Autodesk Fusion 360 part; units mm, degrees
note: some values were not read from the file. Set by a fixed rule: the direction of a hole.
(part 2 of 4)
sketch "草图3" plane through (0, 0, 16.2) normal (0, 0, 1) x (-1, 0, 0)
  line L0 (-5, -22) -> (0, -17)
  line L1 (0, -17) -> (0, -5)
  line L2 (0, -5) -> (-5, 0)
  line L3 (-5, 0) -> (-17, 0)
  line L4 (-17, 0) -> (-22, -5)
  line L5 (-22, -5) -> (-22, -17)
  line L6 (-22, -17) -> (-17, -22)
  line L7 (-17, -22) -> (-5, -22)
  circle A0 centre (-11, -11) radius 9
  dimension "d13" = 18
  dimension "d14" = 11
  dimension "d15" = 11
  measures "d13" diameter of A0
  measures "d14" distance of L7 A0.centre
  measures "d15" distance of L5 A0.centre
extrude "拉伸3" add sketch "草图3" along normal blind 5.5 contours A0
fillet "圆角4" radius 1 1 edges at (19.3909, 7.7455, 16.2)
chamfer "倒角1" distance 2 angle 45 8 edges at (11, 0, 16.2) (19.5, 2.5, 16.2) (22, 11, 16.2) (19.5, 19.5, 16.2) (2.5, 2.5, 16.2) (0, 11, 16.2) (2.5, 19.5, 16.2) (11, 22, 16.2)
sketch "草图4" plane through (0, 0, 0) normal (0, 0, -1) x (1, 0, 0)
  arc A0 (17, -22) -> (22, -17) centre (17, -17) ccw
  line L0 (22, -17) -> (22, -5)
  arc A1 (22, -5) -> (17, 0) centre (17, -5) ccw
  line L1 (17, 0) -> (5, 0)
  arc A2 (5, 0) -> (0, -5) centre (5, -5) ccw
  line L2 (0, -5) -> (0, -17)
  arc A3 (0, -17) -> (5, -22) centre (5, -17) ccw
  line L3 (5, -22) -> (17, -22)
  circle A4 centre (4.75, -17) radius 1.2
  circle A5 centre (17.25, -17) radius 1.2
  dimension "d23" = 2.4
  dimension "d24" = 2.4
  dimension "d25" = 12.5
  dimension "d26" = 4.75
  dimension "d27" = 5
  measures "d23" diameter of A4
  measures "d24" diameter of A5
  measures "d25" distance of A4.centre A5.centre
  measures "d26" distance of L2 A4.centre
  measures "d27" distance of L3 A4.centre
extrude "拉伸4" cut sketch "草图4" against normal blind 5 contours A4 | A5
sketch "草图5" plane through (0, 0, 0) normal (0, 0, -1) x (1, 0, 0)
  circle A0 centre (4.75, -17) radius 1.2
  circle A1 centre (17.25, -17) radius 1.2
  arc A2 (17, -22) -> (22, -17) centre (17, -17) ccw
  line L0 (22, -17) -> (22, -5)
  arc A3 (22, -5) -> (17, 0) centre (17, -5) ccw
  line L1 (17, 0) -> (5, 0)
  arc A4 (5, 0) -> (0, -5) centre (5, -5) ccw
  line L2 (0, -5) -> (0, -17)
  arc A5 (0, -17) -> (5, -22) centre (5, -17) ccw
  line L3 (5, -22) -> (17, -22)
  circle A6 centre (11, -14) radius 3.25
  dimension "d30" = 6.5
  dimension "d33" = 8
  measures "d30" diameter of A6
  measures "d33" distance of L3 A6.centre
extrude "拉伸5" add sketch "草图5" along normal blind 3 contours A6

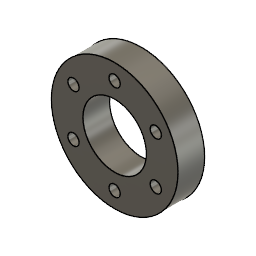
design "输出轴垫块---2"
part number: 2026-07-22-15-46-42-042
Autodesk Fusion 360 part; units mm, degrees
sketch "草图1" plane through (0, 0, 0) normal (0, 0, 1) x (1, 0, 0)
  circle A0 centre (6.115, -10.5915) radius 1.7
  circle A1 centre (-12.23, 0) radius 1.7
  arc A2 (-10.145, 12.6301) -> (-10.3229, 9.3593) centre (-8.7673, 10.9149) ccw
  circle A3 centre (6.115, 10.5915) radius 1.7
  arc A4 (-1.5064, -8.2546) -> (-2.6915, -5.6961) centre (-3.6314, -7.6852) ccw
  arc A5 (-2.9439, 13.6195) -> (-5.8655, 15.1009) centre (-5.0689, 13.0501) ccw
  line L0 (13.2668, -4.2603) -> (7.9019, -2.8228)
  line L1 (-6.3955, 5.4319) -> (-10.3229, 9.3593)
  circle A6 centre (11.6913, 6.75) radius 1.6
  line L2 (-2.9439, 13.6195) -> (-1.5064, 8.2547)
  arc A7 (6.2787, -0.5171) -> (6.2787, 0.5171) centre (0, 0) ccw
  arc A8 (16.0105, 2.4708) -> (13.2668, 4.2603) centre (13.8362, 2.1352) ccw
  arc A9 (-5.8655, 15.1009) -> (-10.145, 12.6301) centre (0, 0) ccw
  line L3 (7.9019, 2.8227) -> (13.2668, 4.2603)
  circle A10 centre (11.6913, -6.75) radius 1.6
  arc A11 (13.2668, -4.2603) -> (16.0105, -2.4708) centre (13.8362, -2.1352) ccw
  arc A12 (-10.145, -12.6301) -> (-5.8655, -15.1009) centre (0, 0) ccw
  arc A13 (-10.3229, -9.3593) -> (-10.145, -12.6301) centre (-8.7673, -10.9149) ccw
  arc A14 (-3.5872, -5.179) -> (-6.3955, -5.4319) centre (-4.8399, -6.9875) ccw
  circle A15 centre (0, 13.5) radius 1.6
  circle A16 centre (-11.6913, -6.75) radius 1.6
  circle A17 centre (0, 0) radius 4.75
  arc A18 (-2.6915, 5.6961) -> (-3.5872, 5.179) centre (0, 0) ccw
  circle A19 centre (-11.6913, 6.75) radius 1.6
  arc A20 (6.2787, -0.5171) -> (7.9019, -2.8228) centre (8.4713, -0.6977) ccw
  arc A21 (-6.3955, 5.4319) -> (-3.5872, 5.179) centre (-4.8399, 6.9875) ccw
  arc A22 (-3.5872, -5.179) -> (-2.6915, -5.6961) centre (0, 0) ccw
  circle A23 centre (0, -13.5) radius 1.6
  arc A24 (-2.6915, 5.6961) -> (-1.5064, 8.2547) centre (-3.6314, 7.6852) ccw
  circle A25 centre (0, 0) radius 18
  arc A26 (7.9019, 2.8227) -> (6.2787, 0.5171) centre (8.4713, 0.6977) ccw
  line L4 (-1.5064, -8.2546) -> (-2.9439, -13.6195)
  line L5 (-10.3229, -9.3593) -> (-6.3955, -5.4319)
  arc A27 (16.0105, -2.4708) -> (16.0105, 2.4708) centre (0, 0) ccw
  arc A28 (-5.8655, -15.1009) -> (-2.9439, -13.6195) centre (-5.0689, -13.0501) ccw
  dimension "d3" = 36
  dimension "d4" = 3.2
  constraint equal A6 A15
  constraint equal A6 A10
  constraint equal A10 A23
  constraint equal A16 A23
  constraint equal A16 A19
  measures "d3" diameter of A25
  measures "d4" diameter of A15
extrude "拉伸1" add sketch "草图1" along normal blind 7.6 contours A0 | A1 | A2 A5 L1 L2 A9 A18 A21 A24 | A3 | A4 A12 A13 A14 A22 L4 L5 A28 | L0 A7 A8 L3 A11 A20 A26 A27 | A25
sketch "草图2" plane through (0, 0, 7.6) normal (0, 0, 1) x (1, 0, 0)
  circle A0 centre (11.6913, -6.75) radius 1.6
  circle A1 centre (11.6913, 6.75) radius 1.6
  circle A2 centre (-11.6913, 6.75) radius 1.6
  circle A3 centre (0, 13.5) radius 1.6
  circle A4 centre (-11.6913, -6.75) radius 1.6
  circle A5 centre (0, 0) radius 4.75
  circle A6 centre (0, -13.5) radius 1.6
  circle A7 centre (0, 0) radius 18
  circle A8 centre (0, 0) radius 9
  dimension "d5" = 18
  constraint coincident A5.centre A7.centre
  measures "d5" diameter of A8
extrude "拉伸2" cut sketch "草图2" against normal blind 20 contours A8

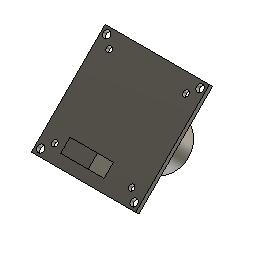
design "New Camera"
part number: 2026-07-08-15-06-55-000
Autodesk Fusion 360 part; units mm, degrees
sketch "sketch 1014" plane through (0, -331.5766, 331.5766) normal (0, -0.707107, 0.707107) x (1, 0, 0)
  line L0 (19, 44) -> (19, 82)
  line L1 (19, 82) -> (-19, 82)
  line L2 (-19, 82) -> (-19, 44)
  line L3 (-19, 44) -> (19, 44)
  circle A0 centre (14, 77) radius 1
  circle A1 centre (17, 80) radius 1.25
  circle A2 centre (-14, 49) radius 1
  circle A3 centre (-17, 80) radius 1.25
  circle A4 centre (-14, 77) radius 1
  circle A5 centre (17, 46) radius 1.25
  circle A6 centre (14, 49) radius 1
  circle A7 centre (-17, 46) radius 1.25
extrude "拉伸1" add sketch "sketch 1014" along normal blind 1.6
sketch "草图1" plane through (0, -331.5766, 331.5766) normal (0, 0.707107, -0.707107) x (-1, 0, 0)
  line L0 (-19, 82) -> (-19, 44)
  line L1 (-19, 44) -> (19, 44)
  line L2 (19, 44) -> (19, 82)
  line L3 (19, 82) -> (-19, 82)
  circle A0 centre (-17, 46) radius 1.25
  circle A1 centre (-14, 77) radius 1
  circle A2 centre (14, 77) radius 1
  circle A3 centre (17, 80) radius 1.25
  circle A4 centre (17, 46) radius 1.25
  circle A5 centre (-14, 49) radius 1
  circle A6 centre (-17, 80) radius 1.25
  circle A7 centre (14, 49) radius 1
  line L4 (-19, 82) -> (19, 44) construction
  line L5 (19, 82) -> (-19, 44) construction
  line L6 (-7, 70) -> (7, 70)
  line L7 (7, 70) -> (7, 56)
  line L8 (7, 56) -> (-7, 56)
  line L9 (-7, 56) -> (-7, 70)
  line L10 (-7, 70) -> (7, 56) construction
  line L11 (7, 70) -> (-7, 56) construction
  line L12 (-7, 63) -> (7, 63) construction
  line L13 (-7, 65.15) -> (-8.85, 65.15)
  arc A8 (-8.85, 65.15) -> (-8.85, 60.85) centre (-8.85, 63) ccw
  line L14 (-8.85, 60.85) -> (-7, 60.85)
  line L15 (0, 70) -> (0, 56) construction
  arc A9 (8.85, 60.85) -> (8.85, 65.15) centre (8.85, 63) ccw
  line L16 (7, 65.15) -> (8.85, 65.15)
  line L17 (8.85, 60.85) -> (7, 60.85)
  point P0 (0, 63)
  point P1 (0, 63)
  point P2 (-11, 63)
  dimension "d359" = 14
  dimension "d360" = 4.3
  dimension "d362" = 11
  constraint coincident L0.start L3.end
  constraint coincident L1.end L2.start
  constraint coincident L2.end L3.start
  constraint coincident L0.end L1.start
  constraint midpoint L4 P1
  constraint horizontal L6
  constraint perpendicular L6 L7
  constraint parallel L6 L8
  constraint parallel L7 L9
  constraint coincident L10 P1
  constraint coincident L11 P1
  constraint coincident P1 P0
  constraint equal L6 L9
  constraint midpoint L9 L12.start
  constraint midpoint L7 L12.end
  constraint coincident L9 L13.start
  constraint perpendicular L9 L13
  constraint tangent L13 A8
  constraint coincident L9 L14.end
  constraint tangent A8 L14
  constraint perpendicular L9 L14
  constraint symmetric L12 L13.start L14.end
  constraint midpoint A8 P2
  constraint midpoint L6 L15.start
  constraint midpoint L8 L15.end
  constraint symmetric L13.start L15 L16.start
  constraint symmetric L13.end L15 A9.end
  constraint symmetric A8.end L15 A9.start
  constraint symmetric A8 L15 A9
  constraint symmetric L14.end L15 L17.end
  measures "d359" distance of L6.end L7.end
  measures "d360" distance of L13 L14
  measures "d362" distance of P1 P2
extrude "拉伸2" add sketch "草图1" along normal blind 3.5 contours L6 L7 L8 L9 | L9 L13 A8 L14 | L7 A9 L16 L17
sketch "草图2" plane through (0, -329.1018, 329.1018) normal (0, 0.707107, -0.707107) x (-1, 0, 0)
  line L0 (-7, 65.15) -> (-8.85, 65.15)
  arc A0 (-8.85, 65.15) -> (-8.85, 60.85) centre (-8.85, 63) ccw
  line L1 (-8.85, 60.85) -> (-7, 60.85)
  line L2 (-7, 60.85) -> (-7, 56)
  line L3 (-7, 56) -> (7, 56)
  line L4 (7, 56) -> (7, 60.85)
  line L5 (7, 60.85) -> (8.85, 60.85)
  arc A1 (8.85, 60.85) -> (8.85, 65.15) centre (8.85, 63) ccw
  line L6 (8.85, 65.15) -> (7, 65.15)
  line L7 (7, 65.15) -> (7, 70)
  line L8 (7, 70) -> (-7, 70)
  line L9 (-7, 70) -> (-7, 65.15)
  line L10 (0, 70) -> (0, 56) construction
  circle A2 centre (0, 63) radius 7
  dimension "d365" = 14
  constraint midpoint L8 L10.start
  constraint midpoint L3 L10.end
  constraint midpoint L10 A2.centre
  measures "d365" diameter of A2
extrude "拉伸3" add sketch "草图2" along normal blind 10.6 contours A2
sketch "草图3" plane through (1.3279, -320.4832, 322.7296) normal (0, 0.707107, -0.707107) x (-1, 0, 0)
  circle A0 centre (1.3279, 61.4116) radius 8.5
  circle A1 centre (1.3279, 61.4116) radius 7 construction
  dimension "d369" = 17
  constraint coincident A0.centre A1.centre
  measures "d369" diameter of A0
extrude "拉伸4" add sketch "草图3" along normal blind 7.3
sketch "草图4" plane through (0, -332.708, 332.708) normal (0, -0.707107, 0.707107) x (1, 0, 0)
  line L0 (-19, 44) -> (19, 44)
  line L1 (19, 44) -> (19, 82)
  line L2 (19, 82) -> (-19, 82)
  line L3 (-19, 82) -> (-19, 44)
  circle A0 centre (14, 49) radius 1
  circle A1 centre (-14, 77) radius 1
  circle A2 centre (17, 46) radius 1.25
  circle A3 centre (-17, 80) radius 1.25
  circle A4 centre (-14, 49) radius 1
  circle A5 centre (-17, 46) radius 1.25
  circle A6 centre (17, 80) radius 1.25
  circle A7 centre (14, 77) radius 1
  line L4 (-5, 52.3) -> (5, 52.3)
  line L5 (5, 52.3) -> (5, 47.5)
  line L6 (5, 47.5) -> (-5, 47.5)
  line L7 (-5, 47.5) -> (-5, 52.3)
  line L8 (0, 44) -> (0, 52.3) construction
  line L9 (-19, 44) -> (19, 44)
  dimension "d1" = 3.5
  dimension "d2" = 4.8
  dimension "d3" = 10
  constraint horizontal L4
  constraint vertical L5
  constraint horizontal L6
  constraint vertical L7
  constraint midpoint L0 L8.start
  constraint midpoint L4 L8.end
  constraint vertical L8
  measures "d1" distance of L6 L9
  measures "d2" distance of L4.start L6.end
  measures "d3" distance of L4.start L4.end
extrude "拉伸5" add sketch "草图4" along normal blind 8.2 contours L4 L5 L6 L7

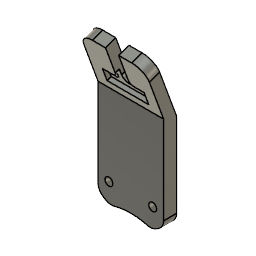
design "Maker Arm 摄像头支架-UW"
part number: 2026-08-07-11-14-49-423
Autodesk Fusion 360 part; units mm, degrees
sketch "草图2" plane through (0, 0, 0) normal (1, 0, 0) x (0, 1, 0)
  line L0 (-6, 73.2538) -> (-6, 0)
  line L1 (0, 71.388) -> (0, 0)
  line L2 (-6, 0) -> (0, 0)
  line L3 (0, 71.388) -> (-9.852, 98.4563)
  line L4 (-9.852, 98.4563) -> (-14.5505, 96.7462)
  line L5 (-14.5505, 96.7462) -> (-6, 73.2538)
  point P0 (-10.2753, 85)
  dimension "d70" = 6
  dimension "d71" = 5
  dimension "d72" = 25
  dimension "d73" = 160
  dimension "d74" = 85
  constraint vertical L0
  constraint vertical L1
  constraint perpendicular L1 L2
  constraint coincident L1.end L2.end
  constraint perpendicular L3 L4
  constraint perpendicular L4 L5
  constraint midpoint L5 P0
  measures "d70" distance of L0.end L1.end
  measures "d71" distance of L3.end L4.end
  measures "d72" distance of L0.start L4.end
  measures "d73" angle of L0 L5
  measures "d74" distance of L2 P0
extrude "拉伸2" add sketch "草图2" along normal mid plane 30
sketch "草图12" plane through (0, -6, 0) normal (0, -1, 0) x (1, 0, 0)
  line L0 (-15, 0) -> (15, 0)
  line L1 (15, 0) -> (15, 73.2538)
  line L2 (15, 73.2538) -> (-15, 73.2538)
  line L3 (-15, 73.2538) -> (-15, 0)
  circle A0 centre (0, 0) radius 28.5
  circle A1 centre (-10, 36) radius 1.8
  circle A2 centre (10, 36) radius 1.8
  line L4 (0, 0) -> (0, 28.5) construction
  dimension "d92" = 57
  dimension "d93" = 3.6
  dimension "d94" = 36
  dimension "d95" = 20
  constraint coincident A0.centre L4.start
  constraint coincident A0 L4.end
  constraint perpendicular L0 L4
  constraint symmetric A1.centre A2.centre L4
  constraint equal A1 A2
  measures "d92" diameter of A0
  measures "d93" diameter of A1
  measures "d94" vertical distance of A0.centre A1.centre
  measures "d95" distance of A1.centre A2.centre
extrude "拉伸13" cut sketch "草图12" against normal up to surface (6 mm away) contours L0 L1 L3 A0 | A1 | A2 picked at (0, 9.5)
chamfer "倒角5" distance 6 angle 45 2 edges at (-15, -3, 24.2332) (15, -3, 24.2332)
fillet "圆角2" radius 5 4 edges at (-9.5942, -3, 26.8366) (9.5942, -3, 26.8366) (-15, -3, 30.2332) (15, -3, 30.2332)
sketch "草图13" plane through (0, 22.9437, 8.3508) normal (0, 0.939693, 0.34202) x (-1, 0, 0)
  line L0 (15, 95.8882) -> (-15, 95.8882)
  line L1 (-15, 95.8882) -> (-15, 67.0828)
  line L2 (-15, 67.0828) -> (15, 67.0828)
  line L3 (15, 67.0828) -> (15, 95.8882)
  line L4 (-3, 95.8882) -> (-3, 79.8882)
  arc A0 (-3, 79.8882) -> (3, 79.8882) centre (0, 79.8882) ccw
  line L5 (3, 79.8882) -> (3, 95.8882)
  line L6 (-6.25, 77.8882) -> (6.25, 77.8882) construction
  line L7 (0, 95.8882) -> (0, 77.8882) construction
  circle A1 centre (-6.25, 77.8882) radius 1.2
  circle A2 centre (6.25, 77.8882) radius 1.2
  line L8 (-11, 72.3882) -> (11, 72.3882) construction
  line L9 (11, 72.3882) -> (11, 94.3882) construction
  line L10 (11, 94.3882) -> (-11, 94.3882) construction
  line L11 (-11, 94.3882) -> (-11, 72.3882) construction
  line L12 (-11, 72.3882) -> (11, 94.3882) construction
  line L13 (11, 72.3882) -> (-11, 94.3882) construction
  point P0 (0, 83.3882)
  dimension "d103" = 3
  dimension "d105" = 2.4
  dimension "d106" = 12.5
  dimension "d107" = 2
  dimension "d109" = 22
  dimension "d110" = 3.5
  dimension "d111" = 12.5
  constraint coincident L0 L4.start
  constraint perpendicular L0 L4
  constraint tangent L4 A0
  constraint tangent A0 L5
  constraint perpendicular L0 L5
  constraint horizontal L6
  constraint midpoint L0 L7.start
  constraint midpoint L6 L7.end
  constraint coincident L6.start A1.centre
  constraint coincident L6.end A2.centre
  constraint equal A1 A2
  constraint vertical L7
  constraint coincident A0.centre L7
  constraint coincident L0 L5.end
  constraint horizontal L8
  constraint perpendicular L8 L9
  constraint parallel L8 L10
  constraint parallel L9 L11
  constraint coincident L12 P0
  constraint coincident L13 P0
  constraint coincident L7 P0
  constraint equal L10 L11
  measures "d103" radius of A0
  measures "d105" diameter of A1
  measures "d106" distance of L6.start L6.end
  measures "d107" distance of A0.centre L6
  measures "d109" distance of L8.start L8.end
  measures "d110" distance of A0.centre P0
  measures "d111" distance of L7.start P0
extrude "拉伸14" cut sketch "草图13" against normal up to surface (5 mm away) contours L0 L4 A0 L5 | A1 | A2
sketch "草图15" plane through (0, 18.2452, 6.6407) normal (0, -0.939693, -0.34202) x (1, 0, 0)
  line L0 (3, 95.8882) -> (3, 79.8882)
  arc A0 (-3, 79.8882) -> (3, 79.8882) centre (0, 79.8882) ccw
  line L1 (-3, 79.8882) -> (-3, 95.8882)
  line L2 (-3, 95.8882) -> (-15, 95.8882)
  line L3 (-15, 95.8882) -> (-15, 70.8882)
  line L4 (-15, 70.8882) -> (15, 70.8882)
  line L5 (15, 70.8882) -> (15, 95.8882)
  line L6 (15, 95.8882) -> (3, 95.8882)
  circle A1 centre (-6.25, 77.8882) radius 1.2
  circle A2 centre (6.25, 77.8882) radius 1.2
  line L7 (-9.5, 80.9882) -> (9.5, 80.9882)
  line L8 (9.5, 80.9882) -> (9.5, 74.7882)
  line L9 (9.5, 74.7882) -> (-9.5, 74.7882)
  line L10 (-9.5, 74.7882) -> (-9.5, 80.9882)
  line L11 (-9.5, 77.8882) -> (9.5, 77.8882) construction
  line L12 (0, 80.9882) -> (0, 74.7882) construction
  dimension "d120" = 6.2
  dimension "d121" = 19
  constraint horizontal L7
  constraint vertical L8
  constraint horizontal L9
  constraint vertical L10
  constraint midpoint L10 L11.start
  constraint midpoint L8 L11.end
  constraint midpoint L7 L12.start
  constraint midpoint L9 L12.end
  constraint coincident A1.centre L11
  constraint symmetric A1.centre A2.centre L12
  measures "d120" distance of L7.start L9.end
  measures "d121" distance of L8.end L9.end
extrude "拉伸16" cut sketch "草图15" against normal blind 2 contours L0 A0 L1 L7 L8 L9 L10
fillet "圆角4" radius 2 2 edges at (-3, -8.5147, 83.0868) (3, -8.5147, 83.0868)
fillet "圆角4" radius 6 2 edges at (-15, -12.2013, 97.6012) (15, -12.2013, 97.6012)

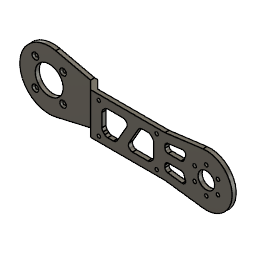
design "L2侧臂-2"
part number: 2026-08-10-10-33-43-885
Autodesk Fusion 360 part; units mm, degrees
sketch "草图1" plane through (0, 0, 0) normal (0, 0, 1) x (1, 0, 0)
  line L0 (0, -20) -> (160, -20)
  arc A0 (160, -20) -> (160, 20) centre (160, 0) ccw
  line L1 (160, 20) -> (0, 20)
  arc A1 (0, 20) -> (0, -20) centre (0, 0) ccw
  line L2 (0, 0) -> (160, 0) construction
  circle A2 centre (0, 0) radius 28.5
  circle A3 centre (160, 0) radius 25
  circle A4 centre (160, 0) radius 8
  circle A5 centre (160, 0) radius 13 construction
  circle A6 centre (160, 13) radius 1.65
  circle A7 centre (148.7417, 6.5) radius 1.65
  circle A8 centre (148.7417, -6.5) radius 1.65
  circle A9 centre (160, -13) radius 1.65
  circle A10 centre (171.2583, -6.5) radius 1.65
  circle A11 centre (171.2583, 6.5) radius 1.65
  line L3 (6.4228, 27.7668) -> (40, 20)
  line L4 (6.4228, -27.7668) -> (40, -20)
  line L5 (156.7702, 24.7905) -> (120, 20)
  line L6 (120, -20) -> (156.7702, -24.7905)
  circle A12 centre (0, 0) radius 19 construction
  circle A13 centre (-13.435, 13.435) radius 1.65
  circle A14 centre (-13.435, -13.435) radius 1.65
  circle A15 centre (13.435, -13.435) radius 1.65
  circle A16 centre (13.435, 13.435) radius 1.65
  line L7 (-13.435, 13.435) -> (0, 0) construction
  line L8 (0, 0) -> (0, 32.5193) construction
  circle A17 centre (0, 0) radius 13.5
  dimension "d1" = 160
  dimension "d2" = 16
  dimension "d3" = 26
  dimension "d4" = 3.3
  dimension "d6" = 360
  dimension "d9" = 57
  dimension "d11" = 40
  dimension "d13" = 20
  dimension "d15" = 38
  dimension "d16" = 20
  dimension "d17" = 3.3
  dimension "d19" = 360
  dimension "d20" = 45
  dimension "d21" = 27
  dimension "d75" = 50
  dimension "d76" = 40
  dimension "d77" = 40
  constraint tangent L0 A0
  constraint tangent A0 L1
  constraint parallel L0 L1
  constraint horizontal L2
  constraint coincident A1.centre L2.start
  constraint concentric A0 A3
  constraint concentric A0 A4
  constraint concentric A0 A5
  constraint coincident A5 A6.centre
  constraint vertical A6.centre A9.centre
  constraint coincident A2 L3.start
  constraint coincident L1 L3.end
  constraint coincident A2 L4.start
  constraint coincident L0 L4.end
  constraint tangent A2 L4
  constraint coincident A3 L5.start
  constraint coincident L1 L5.end
  constraint coincident A3 L6.end
  constraint tangent A3 L5
  constraint tangent A3 L6
  constraint coincident L0 L6.start
  constraint concentric A1 A12
  constraint vertical L0.start L1.end
  constraint tangent A2 L3
  constraint coincident A12 A13.centre
  constraint coincident A13.centre L7.start
  constraint perpendicular L2 L8
  constraint concentric A12 A17
  constraint equal L3 L4
  measures "d1" distance of A0.end L1.end
  measures "d2" diameter of A4
  measures "d3" diameter of A5
  measures "d4" diameter of A6
  measures "d9" diameter of A2
  measures "d11" horizontal distance of A1.centre L3.end
  measures "d13" radius of A0
  measures "d15" diameter of A12
  measures "d16" radius of A1
  measures "d17" diameter of A13
  measures "d20" angle of L7 L8
  measures "d21" diameter of A17
  measures "d75" diameter of A3
  measures "d76" horizontal distance of A0.centre L5.end
  measures "d77" horizontal distance of A0.centre L6.start
extrude "拉伸1" add sketch "草图1" along normal blind 12 contours L0 L1 A2 A3 | L0 A2 L4 | L0 A3 L6 | L0 L1 A1 A2 A13 A14 | L0 L1 A1 A2 A13 A14 | L0 A0 L1 A3 | L0 A0 L1 A3 | L1 A2 L3 | L1 A3 L5
sketch "草图2" plane through (0, 20, 0) normal (0, 1, 0) x (-1, 0, 0)
  line L0 (-120, 0) -> (-40, 0)
  line L1 (-40, 0) -> (-40, 12)
  line L2 (-40, 12) -> (-120, 12)
  line L3 (-120, 12) -> (-120, 0)
  line L4 (29.704, 4) -> (-40, 4)
  line L5 (-40, 4) -> (-40, 12)
  line L6 (-40, 12) -> (29.704, 12)
  line L7 (29.704, 12) -> (29.704, 4)
  line L8 (-120, 0) -> (-190, 0)
  line L9 (-190, 0) -> (-190, 8)
  line L10 (-190, 8) -> (-120, 8)
  line L11 (-120, 8) -> (-120, 0)
  line L12 (-40, 4) -> (-48, 12)
  line L13 (-43.0711, 0) -> (-51.0711, 8)
  line L14 (-51.0711, 8) -> (-120, 8)
  dimension "d24" = 8
  dimension "d25" = 8
  dimension "d26" = 45
  dimension "d27" = 5
  constraint horizontal L4
  constraint vertical L5
  constraint horizontal L6
  constraint vertical L7
  constraint coincident L1.end L2.start
  constraint horizontal L8
  constraint vertical L9
  constraint horizontal L10
  constraint vertical L11
  constraint coincident L0.start L3.end
  constraint coincident L2 L12.end
  constraint coincident L0 L13.start
  constraint parallel L12 L13
  constraint horizontal L14
  measures "d24" distance of L8.end L9.end
  measures "d25" distance of L4.start L6.end
  measures "d26" angle of L0 L12
  measures "d27" distance of L12 L13
extrude "拉伸2" cut sketch "草图2" along normal blind -50 and the other way blind -40 contours L0 L3 L11 L13 L14 | L3 L8 L9 L10 L11 | L1 L2 L5 L12 | L1 L4 L5 L6 L7
sketch "草图3" plane through (0, 0, 12) normal (0, 0, 1) x (1, 0, 0)
  circle A0 centre (171.2583, 6.5) radius 1.65
  circle A1 centre (160, -13) radius 1.65
  circle A2 centre (148.7417, -6.5) radius 1.65
  circle A3 centre (148.7417, 6.5) radius 1.65
  circle A4 centre (171.2583, -6.5) radius 1.65
  circle A5 centre (160, 0) radius 8
  circle A6 centre (160, 13) radius 1.65
  line L0 (48, 20) -> (48, -20)
  line L1 (48, -20) -> (120, -20)
  line L2 (120, -20) -> (156.7702, -24.7905)
  arc A7 (156.7702, -24.7905) -> (156.7702, 24.7905) centre (160, 0) ccw
  line L3 (156.7702, 24.7905) -> (120, 20)
  line L4 (120, 20) -> (48, 20)
  circle A8 centre (160, 0) radius 22 construction
  arc A9 (160, 24.5) -> (138.7824, 12.25) centre (160, 0) ccw
  arc A10 (160, 19.5) -> (160, 24.5) centre (160, 22) ccw
  arc A11 (160, 19.5) -> (143.1125, 9.75) centre (160, 0) ccw
  arc A12 (138.7824, 12.25) -> (143.1125, 9.75) centre (140.9474, 11) ccw
  arc A13 (160, 22) -> (140.9474, 11) centre (160, 0) ccw construction
  line L5 (160, 22) -> (160, 0) construction
  line L6 (160, 0) -> (140.9474, 11) construction
  arc A14 (138.7824, -12.25) -> (160, -24.5) centre (160, 0) ccw
  arc A15 (143.1125, -9.75) -> (138.7824, -12.25) centre (140.9474, -11) ccw
  arc A16 (143.1125, -9.75) -> (160, -19.5) centre (160, 0) ccw
  arc A17 (160, -24.5) -> (160, -19.5) centre (160, -22) ccw
  arc A18 (181.2176, -12.25) -> (181.2176, 12.25) centre (160, 0) ccw
  arc A19 (176.8875, -9.75) -> (181.2176, -12.25) centre (179.0526, -11) ccw
  arc A20 (176.8875, -9.75) -> (176.8875, 9.75) centre (160, 0) ccw
  arc A21 (181.2176, 12.25) -> (176.8875, 9.75) centre (179.0526, 11) ccw
  dimension "d32" = 44
  dimension "d34" = 5
  dimension "d35" = 60
  dimension "d37" = 360
  constraint concentric A5 A8
  constraint tangent A9 A10
  constraint tangent A10 A11
  constraint tangent A11 A12
  constraint tangent A9 A12
  constraint coincident A5.centre A7.centre
  constraint coincident A8 A12.centre
  constraint coincident A10.centre A13.start
  constraint coincident A12.centre A13.end
  measures "d32" diameter of A8
  measures "d34" distance of A9 A11
  measures "d35" angle of L5 L6
sketch "草图4" plane through (0, 0, 12) normal (0, 0, 1) x (1, 0, 0)
  line L0 (48, 20) -> (48, -20)
  line L1 (48, -20) -> (120, -20)
  line L2 (120, -20) -> (156.7702, -24.7905)
  arc A0 (156.7702, -24.7905) -> (156.7702, 24.7905) centre (160, 0) ccw
  line L3 (156.7702, 24.7905) -> (120, 20)
  line L4 (120, 20) -> (48, 20)
  circle A1 centre (148.7417, -6.5) radius 1.65
  circle A2 centre (171.2583, 6.5) radius 1.65
  circle A3 centre (160, -13) radius 1.65
  circle A4 centre (160, 13) radius 1.65
  circle A5 centre (148.7417, 6.5) radius 1.65
  circle A6 centre (171.2583, -6.5) radius 1.65
  circle A7 centre (160, 0) radius 8
  line L5 (56, 15) -> (112, 15) construction
  line L6 (112, 15) -> (112, -15) construction
  line L7 (112, -15) -> (56, -15) construction
  line L8 (56, -15) -> (56, 15) construction
  circle A8 centre (56, 15) radius 1.6
  circle A9 centre (112, 15) radius 1.6
  circle A10 centre (56, -15) radius 1.6
  circle A11 centre (112, -15) radius 1.6
  line L9 (59, -8.1005) -> (59, 8.1005)
  line L10 (109, 8.1005) -> (109, -8.1005)
  line L11 (59, 8.1005) -> (62.8995, 12)
  line L12 (105.1005, 12) -> (109, 8.1005)
  line L13 (105.1005, -12) -> (109, -8.1005)
  line L14 (62.8995, -12) -> (59, -8.1005)
  line L15 (86.3094, 12) -> (72.453, -12)
  line L16 (95.547, 12) -> (81.6906, -12)
  line L17 (62.8995, 12) -> (86.3094, 12)
  line L18 (81.6906, -12) -> (105.1005, -12)
  line L19 (62.8995, 12) -> (86.3094, 12)
  line L20 (95.547, 12) -> (105.1005, 12)
  line L21 (105.1005, -12) -> (81.6906, -12)
  line L22 (72.453, -12) -> (62.8995, -12)
  point P0 (109, -12)
  point P1 (59, -12)
  point P2 (59, 12)
  point P3 (109, 12)
  dimension "d40" = 8
  dimension "d41" = 5
  dimension "d42" = 5
  dimension "d43" = 8
  dimension "d44" = 3.2
  dimension "d56" = 7
  dimension "d60" = 120
  dimension "d61" = 8
  dimension "d64" = 45
  dimension "d65" = 45
  dimension "d66" = 45
  dimension "d67" = 45
  constraint horizontal L5
  constraint vertical L6
  constraint horizontal L7
  constraint vertical L8
  constraint coincident L5.start L8.end
  constraint coincident L5.end L6.start
  constraint coincident L7.end L8.start
  constraint coincident L6.end L7.start
  constraint equal A8 A9
  constraint equal A8 A10
  constraint equal A8 A11
  constraint coincident P2 L9
  constraint coincident P2 L19
  constraint coincident P3 L20
  constraint coincident P3 L10
  constraint coincident P0 L21
  constraint coincident P0 L10
  constraint coincident P1 L22
  constraint coincident P1 L9
  constraint equal L11 L13
  constraint parallel L15 L16
  constraint equal L11 L12
  constraint equal L11 L14
  constraint collinear L19 L20
  constraint collinear L21 L22
  constraint equal L17 L21
  measures "d40" distance of L0 L8
  measures "d41" distance of L4 L5
  measures "d42" distance of L1 L7
  measures "d43" distance of L3.end L6
  measures "d44" diameter of A8
  measures "d56" distance of L5.start L11
  measures "d60" angle of L15 L22
  measures "d61" distance of L15 L16
  measures "d64" angle of L11 L19
  measures "d65" angle of L14 L22
  measures "d66" angle of L12 L20
  measures "d67" angle of L13 L21
extrude "拉伸4" cut sketch "草图4" against normal blind 38 contours A8 | A9 | A10 | A11
extrude "拉伸5" cut sketch "草图4" against normal blind 36 contours L9 L11 L14 L15 L17 L19 L22 | L10 L12 L13 L16 L18 L20 L21
fillet "圆角1" radius 4 12 edges at (105.1005, 12, 10) (86.3094, 12, 10) (62.8995, -12, 10) (72.453, -12, 10) (95.547, 12, 10) (81.6906, -12, 10) (105.1005, -12, 10) (109, 8.1005, 10) (109, -8.1005, 10) (59, -8.1005, 10) (59, 8.1005, 10) (62.8995, 12, 10)
sketch "草图5" plane through (0, 0, 8) normal (0, 0, -1) x (-1, 0, 0)
  circle A0 centre (-112, 15) radius 1.6
  circle A1 centre (-56, -15) radius 1.6
  circle A2 centre (-56, 15) radius 1.6
  circle A3 centre (-112, -15) radius 1.6
  line L0 (-51.0711, 20) -> (-120, 20)
  line L1 (-120, 20) -> (-156.7702, 24.7905)
  arc A4 (-156.7702, 24.7905) -> (-156.7702, -24.7905) centre (-160, 0) ccw
  line L2 (-156.7702, -24.7905) -> (-120, -20)
  line L3 (-120, -20) -> (-51.0711, -20)
  line L4 (-51.0711, -20) -> (-51.0711, 20)
  circle A5 centre (-160, 13) radius 1.65
  circle A6 centre (-171.2583, 6.5) radius 1.65
  circle A7 centre (-148.7417, 6.5) radius 1.65
  circle A8 centre (-148.7417, -6.5) radius 1.65
  circle A9 centre (-171.2583, -6.5) radius 1.65
  circle A10 centre (-160, -13) radius 1.65
  circle A11 centre (-160, 0) radius 8
  line L5 (-88.6188, -12) -> (-103.4437, -12)
  arc A12 (-106.2721, -10.8284) -> (-103.4437, -12) centre (-103.4437, -8) ccw
  line L6 (-106.2721, -10.8284) -> (-107.8284, -9.2721)
  arc A13 (-109, -6.4437) -> (-107.8284, -9.2721) centre (-105, -6.4437) ccw
  line L7 (-109, -6.4437) -> (-109, 6.4437)
  arc A14 (-107.8284, 9.2721) -> (-109, 6.4437) centre (-105, 6.4437) ccw
  line L8 (-107.8284, 9.2721) -> (-106.2721, 10.8284)
  arc A15 (-103.4437, 12) -> (-106.2721, 10.8284) centre (-103.4437, 8) ccw
  line L9 (-103.4437, 12) -> (-97.8564, 12)
  arc A16 (-94.3923, 10) -> (-97.8564, 12) centre (-97.8564, 8) ccw
  line L10 (-94.3923, 10) -> (-85.1547, -6)
  arc A17 (-88.6188, -12) -> (-85.1547, -6) centre (-88.6188, -8) ccw
  line L11 (-79.3812, 12) -> (-64.5563, 12)
  arc A18 (-61.7279, 10.8284) -> (-64.5563, 12) centre (-64.5563, 8) ccw
  line L12 (-61.7279, 10.8284) -> (-60.1716, 9.2721)
  arc A19 (-59, 6.4437) -> (-60.1716, 9.2721) centre (-63, 6.4437) ccw
  line L13 (-59, 6.4437) -> (-59, -6.4437)
  arc A20 (-60.1716, -9.2721) -> (-59, -6.4437) centre (-63, -6.4437) ccw
  line L14 (-60.1716, -9.2721) -> (-61.7279, -10.8284)
  arc A21 (-64.5563, -12) -> (-61.7279, -10.8284) centre (-64.5563, -8) ccw
  line L15 (-64.5563, -12) -> (-70.1436, -12)
  arc A22 (-73.6077, -10) -> (-70.1436, -12) centre (-70.1436, -8) ccw
  line L16 (-73.6077, -10) -> (-82.8453, 6)
  arc A23 (-79.3812, 12) -> (-82.8453, 6) centre (-79.3812, 8) ccw
  circle A24 centre (-112, 15) radius 3.15
  circle A25 centre (-56, 15) radius 3.15
  circle A26 centre (-112, -15) radius 3.15
  circle A27 centre (-56, -15) radius 3.15
  dimension "d72" = 6.3
  constraint concentric A0 A24
  constraint concentric A2 A25
  constraint concentric A3 A26
  constraint concentric A1 A27
  constraint equal A24 A25
  constraint equal A24 A26
  constraint equal A25 A27
  measures "d72" diameter of A24
extrude "拉伸6" cut sketch "草图5" against normal blind 1.5 contours A24 | A25 | A26 | A27
sketch "草图6" plane through (0, 0, 12) normal (0, 0, 1) x (1, 0, 0)
  circle A0 centre (112, 15) radius 1.6
  circle A1 centre (56, -15) radius 1.6
  circle A2 centre (56, 15) radius 1.6
  circle A3 centre (112, -15) radius 1.6
  circle A4 centre (148.7417, -6.5) radius 1.65
  circle A5 centre (171.2583, -6.5) radius 1.65
  circle A6 centre (160, 0) radius 8
  circle A7 centre (160, -13) radius 1.65
  circle A8 centre (160, 13) radius 1.65
  circle A9 centre (171.2583, 6.5) radius 1.65
  circle A10 centre (148.7417, 6.5) radius 1.65
  line L0 (48, 20) -> (48, -20)
  line L1 (48, -20) -> (120, -20)
  line L2 (120, -20) -> (156.7702, -24.7905)
  arc A11 (156.7702, -24.7905) -> (156.7702, 24.7905) centre (160, 0) ccw
  line L3 (156.7702, 24.7905) -> (120, 20)
  line L4 (120, 20) -> (48, 20)
  line L5 (103.4437, -12) -> (88.6188, -12)
  arc A12 (85.1547, -6) -> (88.6188, -12) centre (88.6188, -8) ccw
  line L6 (85.1547, -6) -> (94.3923, 10)
  arc A13 (97.8564, 12) -> (94.3923, 10) centre (97.8564, 8) ccw
  line L7 (97.8564, 12) -> (103.4437, 12)
  arc A14 (106.2721, 10.8284) -> (103.4437, 12) centre (103.4437, 8) ccw
  line L8 (106.2721, 10.8284) -> (107.8284, 9.2721)
  arc A15 (109, 6.4437) -> (107.8284, 9.2721) centre (105, 6.4437) ccw
  line L9 (109, 6.4437) -> (109, -6.4437)
  arc A16 (107.8284, -9.2721) -> (109, -6.4437) centre (105, -6.4437) ccw
  line L10 (107.8284, -9.2721) -> (106.2721, -10.8284)
  arc A17 (103.4437, -12) -> (106.2721, -10.8284) centre (103.4437, -8) ccw
  line L11 (64.5563, 12) -> (79.3812, 12)
  arc A18 (82.8453, 6) -> (79.3812, 12) centre (79.3812, 8) ccw
  line L12 (82.8453, 6) -> (73.6077, -10)
  arc A19 (70.1436, -12) -> (73.6077, -10) centre (70.1436, -8) ccw
  line L13 (70.1436, -12) -> (64.5563, -12)
  arc A20 (61.7279, -10.8284) -> (64.5563, -12) centre (64.5563, -8) ccw
  line L14 (61.7279, -10.8284) -> (60.1716, -9.2721)
  arc A21 (59, -6.4437) -> (60.1716, -9.2721) centre (63, -6.4437) ccw
  line L15 (59, -6.4437) -> (59, 6.4437)
  arc A22 (60.1716, 9.2721) -> (59, 6.4437) centre (63, 6.4437) ccw
  line L16 (60.1716, 9.2721) -> (61.7279, 10.8284)
  arc A23 (64.5563, 12) -> (61.7279, 10.8284) centre (64.5563, 8) ccw
  arc A24 (143.1879, 14.9534) -> (143.1879, -14.9534) centre (160, 0) ccw
  line L17 (143.1879, 14.9534) -> (120, 11.9324)
  line L18 (120, 11.9324) -> (120, -11.9324)
  line L19 (120, -11.9324) -> (143.1879, -14.9534)
  line L20 (160, 0) -> (105.4261, 0) construction
  line L21 (137.8584, 4) -> (120, 4)
  line L22 (120, -4) -> (137.8584, -4)
  dimension "d79" = 8
  dimension "d80" = 8
  dimension "d81" = 8
  dimension "d82" = 22.5
  dimension "d83" = 8
  dimension "d84" = 4
  constraint coincident A6.centre A11.centre
  constraint parallel L3 L17
  constraint parallel L2 L19
  constraint vertical L18
  constraint perpendicular L18 L20
  constraint coincident A24 L21.start
  constraint coincident L18 L21.end
  constraint perpendicular L18 L21
  constraint coincident L18 L22.start
  constraint coincident A24 L22.end
  constraint perpendicular L18 L22
  measures "d79" distance of A0.centre L18
  measures "d80" distance of L3 L17
  measures "d81" distance of L2 L19
  measures "d82" radius of A24
  measures "d83" distance of L21 L22
  measures "d84" distance of L20 L21
extrude "拉伸7" cut sketch "草图6" against normal blind 37 contours A24 L17 L18 L21 | A24 L18 L19 L22
fillet "圆角2" radius 3 8 edges at (120, 4, 10) (120, 11.9324, 10) (143.1879, 14.9534, 10) (137.8584, 4, 10) (137.8584, -4, 10) (120, -4, 10) (120, -11.9324, 10) (143.1879, -14.9534, 10)
sketch "草图7" plane through (0, 0, 4) normal (0, 0, 1) x (1, 0, 0)
  line L0 (6.4228, -27.7668) -> (40, -20)
  line L1 (40, -20) -> (40, 20)
  line L2 (40, 20) -> (6.4228, 27.7668)
  arc A0 (6.4228, 27.7668) -> (6.4228, -27.7668) centre (0, 0) ccw
  circle A1 centre (13.435, -13.435) radius 1.65
  circle A2 centre (-13.435, 13.435) radius 1.65
  circle A3 centre (13.435, 13.435) radius 1.65
  circle A4 centre (-13.435, -13.435) radius 1.65
  circle A5 centre (0, 0) radius 13.5
hole "孔1" at (-13.435, 13.435, 4) at (13.435, 13.435, 4) at (-13.435, -13.435, 4) at (13.435, -13.435, 4) direction (0, 0, -1) diameter 3.3 depth 8 tip angle 180 countersink diameter 6.3 countersink angle 90

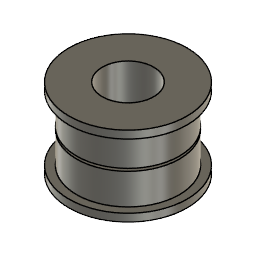
design "MF84ZZ 法兰轴承 4 8 3"
part number: 2026-07-21-18-29-33-284
Autodesk Fusion 360 part; units mm, degrees
sketch "草图2" plane through (0, 0, 0) normal (0, 1, 0) x (1, 0, 0)
  line L0 (0, 0) -> (0, -3.7317) construction
  line L1 (-2, -0.1) -> (-4, -0.1)
  line L2 (-4, -0.1) -> (-4, -2.5)
  line L3 (-4, -2.5) -> (-4.6, -2.5)
  line L4 (-4.6, -2.5) -> (-4.6, -3.1)
  line L5 (-4.6, -3.1) -> (-2, -3.1)
  line L6 (-2, -3.1) -> (-2, -0.1)
  line L7 (4, -0.1) -> (4, -2.5) construction
  line L8 (4.6, -2.5) -> (4.6, -3.1) construction
  line L9 (2, -0.1) -> (4, -0.1) construction
  line L10 (4.6, -3.1) -> (2, -3.1) construction
  line L11 (2, -3.1) -> (2, -0.1) construction
  line L12 (4, -2.5) -> (4.6, -2.5) construction
  dimension "d1" = 4
  dimension "d2" = 8
  dimension "d3" = 9.2
  dimension "d4" = 0.6
  dimension "d5" = 3
  dimension "d7" = 0.1
  constraint coincident L0.start origin
  constraint vertical L0
  constraint horizontal L1
  constraint perpendicular L1 L2
  constraint perpendicular L2 L3
  constraint perpendicular L3 L4
  constraint perpendicular L4 L5
  constraint perpendicular L5 L6
  constraint symmetric L0 L1.end L7.start
  constraint symmetric L0 L2.end L7.end
  constraint symmetric L0 L3.end L8.start
  constraint symmetric L0 L4.end L8.end
  constraint symmetric L0 L5.end L10.end
  constraint symmetric L0 L1.start L9.start
  measures "d1" distance of L6 L11
  measures "d2" distance of L2 L7
  measures "d3" distance of L4 L8
  measures "d4" distance of L3.end L4.end
  measures "d5" distance of L1 L5
  measures "d7" distance of L0.start L1
revolve "旋转1" add sketch "草图2" angle 360 about axis through (0, 0, 0) along (0, 0, 1) makes body 1
mirror "镜像1" about plane through (0, 0, 0) normal (0, 0, 1) of bodies 1 makes body 2

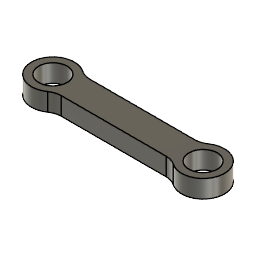
design "连杆"
part number: 2026-07-22-11-51-48-530
Autodesk Fusion 360 part; units mm, degrees
sketch "草图1" plane through (0, 0, 0) normal (0, 0, 1) x (1, 0, 0)
  line L0 (0, 0) -> (-21, 0) construction
  line L1 (0, 4) -> (-16.5279, 4)
  arc A0 (-16.5279, 4) -> (-16.5279, -4) centre (-21, 0) ccw
  line L2 (-16.5279, -4) -> (0, -4)
  line L3 (0, 4) -> (0, -4) construction
  circle A1 centre (-21, 0) radius 3.975
  line L4 (0, 4) -> (16.5279, 4)
  line L5 (16.5279, -4) -> (0, -4)
  arc A2 (16.5279, -4) -> (16.5279, 4) centre (21, 0) ccw
  circle A3 centre (21, 0) radius 3.975
  circle A4 centre (21, 0) radius 4.6 construction
  dimension "d1" = 7.95
  dimension "d2" = 6
  dimension "d3" = 9.2
  dimension "d4" = 8
  dimension "d5" = 42
  constraint coincident L0.start origin
  constraint coincident L0.end A0.centre
  constraint horizontal L2
  constraint perpendicular L2 L3
  constraint coincident L0.start L3
  constraint symmetric L0 L1.end A0.end
  constraint concentric A0 A1
  constraint horizontal L1
  constraint symmetric L1.start L3 L4.start
  constraint symmetric L1.end L3 L4.end
  constraint symmetric A0.end L3 L5.start
  constraint symmetric A0 L3 A2
  constraint symmetric L2.end L3 L5.end
  constraint symmetric L3 A1 A3
  constraint concentric A3 A4
  constraint horizontal L0
  measures "d1" diameter of A1
  measures "d2" radius of A0
  measures "d3" diameter of A4
  measures "d4" distance of L1 L2
  measures "d5" distance of L0.end A2.centre
extrude "拉伸1" add sketch "草图1" along normal blind 5
fillet "圆角1" radius 5 4 edges at (-16.5279, -4, 2.5) (16.5279, -4, 2.5) (16.5279, 4, 2.5) (-16.5279, 4, 2.5)
chamfer "倒角1" [suppressed]

design "底板cnc"
part number: 2026-07-22-15-24-34-429
Autodesk Fusion 360 part; units mm, degrees
sketch "草图1" plane through (0, 0, 0) normal (1, 0, 0) x (0, 0, -1)
  line L0 (75, 40) -> (-75, 40)
  line L1 (-75, 40) -> (-75, -40)
  line L2 (-75, -40) -> (75, -40)
  line L3 (75, 40) -> (-75, -40) construction
  line L4 (-75, 40) -> (75, -40) construction
  line L5 (-65, -30) -> (65, -30) construction
  line L6 (65, -30) -> (65, 30) construction
  line L7 (65, 30) -> (-65, 30) construction
  line L8 (-65, 30) -> (-65, -30) construction
  circle A0 centre (-65, 30) radius 2.6
  line L9 (52, -7.8846) -> (-41, -7.8846) construction
  line L10 (-41, -7.8846) -> (-41, 10) construction
  line L11 (-41, 10) -> (52, 10) construction
  line L12 (52, 10) -> (52, -7.8846) construction
  line L13 (-41, -7.8846) -> (52, 10) construction
  circle A1 centre (-41, 10) radius 1.65
  circle A2 centre (41, 10) radius 1.65
  circle A3 centre (-41, -10) radius 1.65
  circle A4 centre (41, -10) radius 1.65
  circle A5 centre (0, 0) radius 19 construction
  circle A6 centre (-13.435, 13.435) radius 1.6
  line L14 (0, 0) -> (0, 19) construction
  line L15 (-13.435, 13.435) -> (0, 0) construction
  circle A7 centre (-13.435, -13.435) radius 1.6
  circle A8 centre (13.435, -13.435) radius 1.6
  circle A9 centre (13.435, 13.435) radius 1.6
  circle A10 centre (45, 30) radius 2.6
  circle A11 centre (-65, -70) radius 2.6
  circle A12 centre (45, -70) radius 2.6
  line L16 (75, -40) -> (75, 40)
  line L17 (30, -30) -> (-30, -30) construction
  line L18 (-30, -30) -> (-30, 30) construction
  line L19 (-30, 30) -> (30, 30) construction
  line L20 (30, 30) -> (30, -30) construction
  line L21 (30, -30) -> (-30, 30) construction
  line L22 (-30, -30) -> (30, 30) construction
  circle A13 centre (-30, 30) radius 1.6
  circle A14 centre (30, 30) radius 1.6
  circle A15 centre (-30, -30) radius 1.6
  circle A16 centre (30, -30) radius 1.6
  dimension "d1" = 150
  dimension "d2" = 80
  dimension "d3" = -10
  dimension "d4" = 5.2
  dimension "d15" = 3.3
  dimension "d18" = 82
  dimension "d19" = -20
  dimension "d22" = 38
  dimension "d23" = 3.2
  dimension "d26" = 360
  dimension "d29" = 110
  dimension "d30" = -100
  dimension "d52" = 80
  dimension "d55" = 10
  dimension "d68" = 60
  dimension "d69" = 60
  dimension "d70" = 3.2
  dimension "d81" = 93
  dimension "d82" = 34
  dimension "d86" = 10
  constraint horizontal L0
  constraint perpendicular L0 L1
  constraint parallel L0 L2
  constraint coincident L3 A5.centre
  constraint coincident L4 A5.centre
  constraint coincident A5.centre L14.start
  constraint coincident L7.end L8.start
  constraint horizontal L9
  constraint perpendicular L9 L10
  constraint parallel L10 L12
  constraint coincident L13 A5.centre
  constraint coincident L10.end L11.start
  constraint coincident A5 A6.centre
  constraint coincident A5 L14.end
  constraint vertical L14
  constraint coincident A6.centre L15.start
  constraint perpendicular L0 L16
  constraint horizontal L11
  constraint horizontal A6.centre A9.centre
  constraint horizontal L17
  constraint perpendicular L17 L18
  constraint parallel L17 L19
  constraint parallel L18 L20
  constraint coincident L21 A5.centre
  constraint coincident L22 A5.centre
  constraint coincident L18.end L19.start
  constraint coincident L19.end L20.start
  constraint coincident L17.end L18.start
  constraint coincident L17.start L20.end
  constraint equal A13 A14
  constraint equal A13 A15
  constraint equal A13 A16
  measures "d1" distance of L0.start L0.end
  measures "d2" distance of L0.start L2.end
  measures "d4" diameter of A0
  measures "d15" diameter of A1
  measures "d22" diameter of A5
  measures "d23" diameter of A6
  measures "d52" distance of L0.end L1.end
  measures "d55" distance of L6 L16
  measures "d68" distance of L18.end L19.end
  measures "d69" distance of L17.end L18.end
  measures "d70" diameter of A13
  measures "d81" distance of L9.start L9.end
  measures "d82" distance of L1 L10
  measures "d86" distance of L11 A5.centre
extrude "拉伸1" add sketch "草图1" along normal blind 6 contours L0 L1 L2 L16 | A0 | A10 | A13 | A14 | A15 | A16
fillet "圆角1" radius 10 4 edges at (3, 40, 75) (3, -40, 75) (3, -40, -75) (3, 40, -75)
sketch "草图6" plane through (0, 0, 0) normal (-1, 0, 0) x (0, 0, 1)
  arc A0 (-65, 40) -> (-75, 30) centre (-65, 30) ccw
  line L0 (-75, 30) -> (-75, -30)
  arc A1 (-75, -30) -> (-65, -40) centre (-65, -30) ccw
  line L1 (-65, -40) -> (65, -40)
  arc A2 (65, -40) -> (75, -30) centre (65, -30) ccw
  line L2 (75, -30) -> (75, 30)
  arc A3 (75, 30) -> (65, 40) centre (65, 30) ccw
  line L3 (65, 40) -> (-65, 40)
  circle A4 centre (41, 10) radius 1.65
  circle A5 centre (-41, 10) radius 1.65
  circle A6 centre (41, -10) radius 1.65
  circle A7 centre (-41, -10) radius 1.65
  circle A8 centre (13.435, 13.435) radius 1.6
  circle A9 centre (13.435, -13.435) radius 1.6
  circle A10 centre (-13.435, 13.435) radius 1.6
  circle A11 centre (-13.435, -13.435) radius 1.6
hole "孔6" at (0, 13.435, -13.435) at (0, 13.435, 13.435) at (0, -13.435, -13.435) at (0, -13.435, 13.435) at (0, 10, -41) at (0, -10, -41) at (0, 10, 41) at (0, -10, 41) direction (1, 0, 0) diameter 3.3 depth 10 tip angle 180 countersink diameter 6.5 countersink angle 90
sketch "草图7" plane through (0, 0, 0) normal (-1, 0, 0) x (0, 0, 1)
  arc A0 (-65, 40) -> (-75, 30) centre (-65, 30) ccw
  line L0 (-75, 30) -> (-75, -30)
  arc A1 (-75, -30) -> (-65, -40) centre (-65, -30) ccw
  line L1 (-65, -40) -> (65, -40)
  arc A2 (65, -40) -> (75, -30) centre (65, -30) ccw
  line L2 (75, -30) -> (75, 30)
  arc A3 (75, 30) -> (65, 40) centre (65, 30) ccw
  line L3 (65, 40) -> (-65, 40)
  circle A4 centre (13.435, -13.435) radius 3.25
  circle A5 centre (13.435, 13.435) radius 3.25
  circle A6 centre (-13.435, 13.435) radius 3.25
  circle A7 centre (-13.435, -13.435) radius 3.25
  circle A8 centre (-41, 10) radius 4
  circle A9 centre (41, 10) radius 4
  circle A10 centre (41, -10) radius 4
  circle A11 centre (-41, -10) radius 4
  circle A12 centre (41, -10) radius 3.25
  circle A13 centre (-41, -10) radius 3.25
  circle A14 centre (-41, 10) radius 3.25
  circle A15 centre (41, 10) radius 3.25
  dimension "d83" = 8
  constraint equal A8 A9
  constraint equal A8 A11
  constraint equal A9 A10
  measures "d83" diameter of A8

design "J5-J6-In"
part number: 2026-08-07-17-06-13-962
Autodesk Fusion 360 part; units mm, degrees
sketch "草图1" plane through (0, 0, 0) normal (0, 0, 1) x (1, 0, 0)
  line L0 (-28.5, 0) -> (28.5, 0)
  line L1 (0, 30) -> (0, 0) construction
  line L2 (-28.5, 0) -> (-28.5, 16)
  line L3 (-28.5, 16) -> (-15.6964, 38.8105)
  arc A0 (15.6964, 38.8105) -> (-15.6964, 38.8105) centre (0, 30) ccw
  line L4 (15.6964, 38.8105) -> (28.5, 16)
  line L5 (28.5, 16) -> (28.5, 0)
  circle A1 centre (0, 30) radius 9
  circle A2 centre (0, 30) radius 13.5 construction
  circle A3 centre (-6.75, 18.3087) radius 1.6
  circle A4 centre (6.75, 18.3087) radius 1.6
  circle A5 centre (13.5, 30) radius 1.6
  circle A6 centre (6.75, 41.6913) radius 1.6
  circle A7 centre (-6.75, 41.6913) radius 1.6
  circle A8 centre (-13.5, 30) radius 1.6
  line L6 (-28.5, 7) -> (28.5, 7)
  dimension "d1" = 57
  dimension "d2" = 30
  dimension "d3" = 16
  dimension "d4" = 18
  dimension "d5" = 27
  dimension "d6" = 18
  dimension "d7" = 3.2
  dimension "d9" = 360
  dimension "d10" = 7
  constraint horizontal L0
  constraint midpoint L0 L1.end
  constraint vertical L1
  constraint coincident L1.end origin
  constraint perpendicular L0 L2
  constraint tangent L3 A0
  constraint tangent A0 L4
  constraint perpendicular L0 L5
  constraint concentric A0 A1
  constraint concentric A1 A2
  constraint coincident L1.start A0.centre
  constraint symmetric L1 L2.end L4.end
  constraint coincident A2 A3.centre
  constraint symmetric L1 A3.centre A4.centre
  constraint coincident L2 L6.start
  constraint coincident L5 L6.end
  constraint perpendicular L5 L6
  measures "d1" distance of L0.start L0.end
  measures "d2" vertical distance of L1.end L1.start
  measures "d3" distance of L0.start L2.end
  measures "d4" radius of A0
  measures "d5" diameter of A2
  measures "d6" diameter of A1
  measures "d7" diameter of A3
  measures "d10" distance of L0 L6
extrude "拉伸1" add sketch "草图1" against normal blind 8
sketch "草图2" plane through (0, 0, 0) normal (0, -1, 0) x (1, 0, 0)
  line L0 (28.5, 0) -> (-28.5, 0)
  line L1 (-28.5, 0) -> (-28.5, -8)
  line L2 (28.5, -8) -> (28.5, 0)
  line L3 (-28.5, -4) -> (28.5, -4) construction
  circle A0 centre (-22, -4) radius 1.25
  circle A1 centre (0, -4) radius 1.25
  circle A2 centre (22, -4) radius 1.25
  line L4 (0, 0) -> (0, -8) construction
  line L5 (-28.5, -8) -> (28.5, -8)
  dimension "d15" = 44
  dimension "d16" = 2.5
  constraint midpoint L1 L3.start
  constraint midpoint L2 L3.end
  constraint coincident L3 A0.centre
  constraint midpoint L3 A1.centre
  constraint coincident L3 A2.centre
  constraint coincident L4.start origin
  constraint equal A0 A1
  constraint equal A1 A2
  constraint symmetric A0.centre A2.centre L4
  measures "d15" distance of A0.centre A2.centre
  measures "d16" diameter of A0
extrude "拉伸3" cut sketch "草图2" against normal blind 5 contours A0 | A1 | A2
fillet "圆角1" radius 8 2 edges at (28.5, 16, -4) (-28.5, 16, -4)